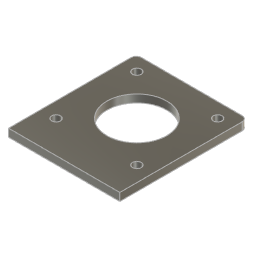
nema mount (Autodesk Fusion 360 archive; units mm, degrees)
design "cr6 nema"
Autodesk Fusion 360 part; units mm, degrees
sketch "Sketch1" plane through (0, 0, 0) normal (0, 0, 1) x (1, 0, 0)
  line L0 (0, 0) -> (42.7, 0)
  line L1 (42.7, 0) -> (42.7, 49)
  line L2 (42.7, 49) -> (0, 49)
  line L3 (0, 49) -> (0, 0)
  circle A0 centre (21.35, 27.9) radius 11.5
  circle A1 centre (5.85, 43.4) radius 1.7
  line L4 (21.35, 49) -> (21.35, 0) construction
  circle A2 centre (5.85, 12.4) radius 1.7
  circle A3 centre (36.85, 43.4) radius 1.7
  circle A4 centre (36.85, 12.4) radius 1.7
  dimension "d1" = 49
  dimension "d2" = 42.7
  dimension "d3" = 9.6
  dimension "d4" = 15.5
  dimension "d5" = 15.5
  dimension "d6" = 3.4
  dimension "d9" = 31
  dimension "d10" = 31
  dimension "d11" = 23
  constraint horizontal L0
  constraint vertical L1
  constraint horizontal L2
  constraint vertical L3
  constraint coincident L0.start L3.end
  constraint midpoint L2 L4.start
  constraint midpoint L0 L4.end
  measures "d1" distance of L0.start L2.end
  measures "d2" distance of L1.end L2.end
  measures "d3" distance of L2 A0
  measures "d4" distance of A1.centre L4
  measures "d5" vertical distance of A0.centre A1.centre
  measures "d6" diameter of A1
  measures "d11" diameter of A0
extrude "Extrude1" add sketch "Sketch1" along normal blind 3
fillet "Fillet1" radius 2 2 edges at (0, 49, 1.5) (42.7, 49, 1.5)
